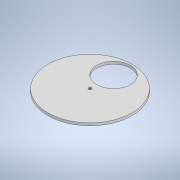
# Autodesk Inventor part: Rotator_(3mm)
Saved by Autodesk Inventor 2020 (Build 240168000, 168)
## iProperties
Created: 2020-12-15
Part Number: Rotator_(3mm)
Material: Generic
Document SubType Name: Modeling
Designer: moham
Density: 1 g/cm^3
Appearance: Default
Author: moham
Autodesk Inventor part; units mm, degrees
ref_plane "YZ Plane" through (0, 0, 0) normal (1, 0, 0) x (0, 1, 0)
ref_plane "XZ Plane" through (0, 0, 0) normal (0, 1, 0) x (-1, 0, 0)
ref_plane "XY Plane" through (0, 0, 0) normal (0, 0, 1) x (1, 0, 0)
sketch "Sketch1" plane through (0, 0, 0) normal (0, 1, 0) x (-1, 0, 0)
  circle A0 centre (0, 0) radius 50
  circle A1 centre (0, -28) radius 20
  circle A2 centre (0, 0) radius 1.7
  dimension "d0" = 100
  dimension "d11" = 40
  dimension "d12" = 3.4
  dimension "d13" = 28
  constraints: 3 centre point, 2 coincident
  measures "d0" diameter of A0
  measures "d11" diameter of A1
  measures "d12" diameter of A2
  measures "d13" distance of point (0, 0) A1.centre
extrude "Extrusion3" add sketch "Sketch1" along normal blind 3
body "Solid2"
